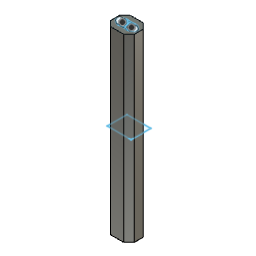
Tennis handle (Autodesk Fusion 360 design; units mm, degrees)
Autodesk Fusion 360 part; units mm, degrees
sketch "Sketch1" plane through (0, 0, 0) normal (0, 0, 1) x (1, 0, 0)
  line L0 (-15, 15) -> (14, 15)
  line L1 (14, 15) -> (14, -9)
  line L2 (14, -9) -> (-15, -9)
  line L3 (-15, -9) -> (-15, 15)
  dimension "d14" = 29
  dimension "d15" = 24
  constraint horizontal L0
  constraint vertical L1
  constraint horizontal L2
  constraint vertical L3
  measures "d14" distance of L0.start L0.end
  measures "d15" distance of L0.start L2.end
extrude "Extrude1" add sketch "Sketch1" along normal blind 220
move_body "Align4" bodies 1 to x (1, 0, 0) y (0, 1, 0) z (0, 0, 1) at (0.5, -3, -110)
chamfer "Chamfer1" distance 6.5 distance2 6.5 1 edges at (14.5, -12, 0) measured on face at (4.8333, -12, -36.6667)
chamfer "Chamfer2" distance 6.5 angle 45 1 edges at (14.5, 12, 0)
chamfer "Chamfer3" distance 6.5 angle 45 1 edges at (-14.5, -12, 0)
chamfer "Chamfer4" distance 6.5 angle 45 1 edges at (-14.5, 12, 0)
sketch "Sketch2" plane through (0, 0, 0) normal (0, 0, 1) x (1, 0, 0)
  circle A0 centre (-9, 0) radius 3.5
  circle A1 centre (9, 0) radius 3.5
  dimension "d10" = 7
  dimension "d11" = 7
  measures "d10" diameter of A0
  measures "d11" diameter of A1
extrude "Extrude2" cut sketch "Sketch2" along normal blind 220 and the other way blind 1100
sketch "Sketch4" plane through (0, 0, 110) normal (0, 0, 1) x (-1, 0, 0)
  circle A0 centre (9, 0) radius 3.5
  circle A1 centre (-9, 0) radius 3.5
  line L0 (8, -12) -> (14.5, -5.5)
  line L1 (14.5, -5.5) -> (14.5, 5.5)
  line L2 (14.5, 5.5) -> (8, 12)
  line L3 (8, 12) -> (-8, 12)
  line L4 (-8, 12) -> (-14.5, 5.5)
  line L5 (-14.5, 5.5) -> (-14.5, -5.5)
  line L6 (-14.5, -5.5) -> (-8, -12)
  line L7 (-8, -12) -> (8, -12)
  line L8 (5.5, -5) -> (-5.5, -5)
  line L9 (5.5, 5) -> (-5.5, 5)
  line L10 (4, -2) -> (-4, -2)
  line L11 (-4, -2) -> (-4, -5)
  line L12 (-4, -5) -> (4, -5)
  line L13 (4, -5) -> (4, -2)
  line L14 (5.5, -5) -> (5.5, 5)
  line L15 (-5.5, -5) -> (-5.5, 5)
  circle A2 centre (9, 0) radius 3.5
  circle A3 centre (-9, 0) radius 3.5
  circle A4 centre (5.5, 0) radius 5.5
  circle A5 centre (-5.5, 0) radius 5.5
  dimension "d24" = 8
  dimension "d27" = 3
  dimension "d28" = 7
  dimension "d29" = 7
  dimension "d30" = 11
  dimension "d31" = 11
  constraint parallel L7 L8
  constraint horizontal L10
  constraint vertical L11
  constraint horizontal L12
  constraint vertical L13
  constraint perpendicular L9 L14
  constraint perpendicular L9 L15
  constraint midpoint L14 A4.centre
  constraint midpoint L15 A5.centre
  measures "d24" distance of L10.start L10.end
  measures "d27" distance of L10.start L12.end
  measures "d28" diameter of A2
  measures "d29" diameter of A3
  measures "d30" diameter of A4
  measures "d31" diameter of A5
extrude "Extrude3" cut sketch "Sketch4" against normal blind 70 contours A0 A2 A4 | A0 L9 L14 A2 A4 | A0 L8 L12 L14 A2 A4 | L8 L9 L10 L13 L14 A4 | L9 A4 A5 | L8 L10 L12 L13 A4 | L8 L10 L12 A4 A5 | L8 L9 L10 L11 L15 A5 | A1 L9 L15 A3 A5 | L10 A4 A5 | A1 L8 L12 L15 A3 A5 | L8 L10 L11 L12 A5 | A1 A3 A5 picked at (9.1952, 0.5641) picked at (-9.1566, 0)
extrude "Extrude4" cut sketch "Sketch4" against normal blind 220 contours L8 L10 L12 L13 A4 | L8 L10 L12 A4 A5 | L8 L10 L11 L12 A5
